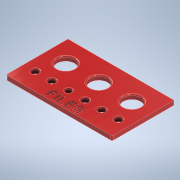
# Autodesk Inventor part: plateForFileSet
Saved by Autodesk Inventor 2021 (Build 250183000, 183)
## iProperties
Created: 2020-03-12
Part Number: plateForFileSet
Material: PET Plastic
Document SubType Name: Modeling
Designer: robst
Density: 1.541 g/cm^3
Appearance: Red
Author: robst
Autodesk Inventor part; units mm, degrees
ref_plane "YZ Plane" through (0, 0, 0) normal (1, 0, 0) x (0, 1, 0)
ref_plane "XZ Plane" through (0, 0, 0) normal (0, 1, 0) x (-1, 0, 0)
ref_plane "XY Plane" through (0, 0, 0) normal (0, 0, 1) x (1, 0, 0)
sketch "Sketch1" plane through (0, 0, 0) normal (0, 1, 0) x (-1, 0, 0)
  line L0 (76.2, 44.45) -> (-76.2, 44.45)
  line L1 (-76.2, 44.45) -> (-76.2, -44.45)
  line L2 (-76.2, -44.45) -> (76.2, -44.45)
  line L3 (76.2, -44.45) -> (76.2, 44.45)
  line L4 (76.2, 44.45) -> (-76.2, -44.45) construction
  line L5 (-76.2, 44.45) -> (76.2, -44.45) construction
  point P0 (0, 0)
  dimension "depth" = 88.9
  dimension "width" = 152.4
  constraints: 12 end point, 2 midpoint, 2 parallel, 1 horizontal, 1 perpendicular
  measures "depth" distance of L2.end L0.start
  measures "width" distance of L1.end L2.end
extrude "Extrusion1" add sketch "Sketch1" against normal blind 6.35
sketch "Sketch4" plane through (0, 0, 0) normal (0, 1, 0) x (1, 0, 0)
  line L0 (-76.2, -44.45) -> (-76.2, 44.45) construction
  line L1 (-76.2, -19.05) -> (76.2, -19.05) construction
  line L2 (76.2, 44.45) -> (76.2, -44.45) construction
  line L3 (-76.2, -44.45) -> (76.2, -44.45) projected
  circle A0 centre (-59.8678, -19.05) radius 4.445
  circle A1 centre (-35.9192, -19.05) radius 4.445
  circle A2 centre (-11.9707, -19.05) radius 3.81
  circle A3 centre (11.9779, -19.05) radius 4.445
  circle A4 centre (35.9265, -19.05) radius 4.445
  line L4 (-76.2, 12.7) -> (76.2, 12.7) construction
  circle A5 centre (-47.625, 12.7) radius 12.7
  circle A6 centre (0, 12.7) radius 12.7
  circle A7 centre (47.625, 12.7) radius 12.7
  circle A8 centre (59.8751, -19.05) radius 4.445
  line L5 (64.3201, -19.05) -> (64.3201, -9.3283) construction
  point P0 (0, 0)
  dimension "file6Hole" = 8.89
  dimension "d16" = 25.4
  dimension "file1Hole" = 8.89
  dimension "gap0" = 11.8872
  dimension "file2Hole" = 8.89
  dimension "gap1" = 23.9486
  dimension "file3Hole" = 7.62
  dimension "gap2" = 23.9486
  dimension "gap3" = 23.9486
  dimension "gap4" = 23.9486
  dimension "file4Hole" = 8.89
  dimension "file5Hole" = 8.89
  dimension "frontToBackRowGap" = 31.75
  dimension "file7Hole" = 25.4
  dimension "file8Hole" = 25.4
  dimension "gap7" = 47.625
  dimension "file9Hole" = 25.4
  dimension "gap8" = 47.625
  dimension "gap6" = 28.575
  dimension "d53" = 28.575
  dimension "file6Gap" = 23.9486
  dimension "d57" = 11.8799
  constraints: 8 centre point, 6 point on line, 4 end point, 2 vertical, 1 horizontal alignment, 1 midpoint, 1 perpendicular, 12 other
  measures "file1Hole" diameter of A0
  measures "gap0" distance edge to line of A0 L0
  measures "file2Hole" diameter of A1
  measures "gap1" distance of A1.centre A0.centre
  measures "file3Hole" diameter of A2
  measures "gap2" distance of A2.centre A1.centre
  measures "gap3" distance of A3.centre A2.centre
  measures "gap4" distance of A4.centre A3.centre
  measures "file4Hole" diameter of A3
  measures "file5Hole" diameter of A4
  measures "file7Hole" diameter of A5
  measures "file8Hole" diameter of A6
  measures "gap7" distance of A6.centre A5.centre
  measures "file9Hole" diameter of A7
  measures "gap8" distance of A7.centre A6.centre
  measures "gap6" distance from line of A5.centre L0
  measures "d53" distance from line of A7.centre L2
  measures "file6Gap" distance of point (59.875, -19.05) A4.centre
  measures "d57" distance of point (76.2, -19.05) L5.start
extrude "Extrusion3" cut sketch "Sketch4" against normal through all
sketch "Sketch8" plane through (0, 0, 0) normal (0, 1, 0) x (1, 0, 0)
  line L0 (76.2, -44.45) -> (-76.2, -44.45) construction
  line L1 (-76.2, -44.45) -> (76.2, -44.45) construction
  line L2 (-23.8464, -41.91) -> (-23.8464, -29.21)
  line L3 (-23.8464, -29.21) -> (-15.1248, -29.21)
  line L4 (-15.1248, -29.21) -> (-15.1248, -31.3589)
  line L5 (-15.1248, -31.3589) -> (-21.2812, -31.3589)
  line L6 (-21.2812, -31.3589) -> (-21.2812, -34.3597)
  line L7 (-21.2812, -34.3597) -> (-15.967, -34.3597)
  line L8 (-15.967, -34.3597) -> (-15.967, -36.5086)
  line L9 (-15.967, -36.5086) -> (-21.2812, -36.5086)
  line L10 (-21.2812, -36.5086) -> (-21.2812, -41.91)
  line L11 (-21.2812, -41.91) -> (-23.8464, -41.91)
  line L12 (-13.092, -41.91) -> (-13.092, -29.21)
  line L13 (-13.092, -29.21) -> (-10.5269, -29.21)
  line L14 (-10.5269, -29.21) -> (-10.5269, -41.91)
  line L15 (-10.5269, -41.91) -> (-13.092, -41.91)
  line L16 (-8.0101, -41.91) -> (-8.0101, -29.3165)
  line L17 (-8.0101, -29.3165) -> (-5.4449, -29.3165)
  line L18 (-5.4449, -29.3165) -> (-5.4449, -39.7611)
  line L19 (-5.4449, -39.7611) -> (0.9341, -39.7611)
  line L20 (0.9341, -39.7611) -> (0.9341, -41.91)
  line L21 (0.9341, -41.91) -> (-8.0101, -41.91)
  line L22 (2.7636, -41.91) -> (2.7636, -29.21)
  line L23 (2.7636, -29.21) -> (12.1821, -29.21)
  line L24 (12.1821, -29.21) -> (12.1821, -31.3589)
  line L25 (12.1821, -31.3589) -> (5.3288, -31.3589)
  line L26 (5.3288, -31.3589) -> (5.3288, -34.1758)
  line L27 (5.3288, -34.1758) -> (11.7078, -34.1758)
  line L28 (11.7078, -34.1758) -> (11.7078, -36.3247)
  line L29 (11.7078, -36.3247) -> (5.3288, -36.3247)
  line L30 (5.3288, -36.3247) -> (5.3288, -39.7611)
  line L31 (5.3288, -39.7611) -> (12.4241, -39.7611)
  line L32 (12.4241, -39.7611) -> (12.4241, -41.91)
  line L33 (12.4241, -41.91) -> (2.7636, -41.91)
  line L34 (13.9439, -37.767) -> (16.4413, -37.525)
  spline S0 degree 2 poles (16.4413, -37.525) (16.6639, -38.7834) (18.0481, -39.9643) (19.2097, -39.9643) knots 0 0 0 1 2 2 2
  spline S1 degree 2 poles (19.2097, -39.9643) (20.4487, -39.9643) (21.7071, -38.9189) (21.7071, -38.2123) knots 0 0 0 1 2 2 2
  spline S2 degree 2 poles (21.7071, -38.2123) (21.7071, -37.7573) (21.1747, -37.1281) (20.5165, -36.8958) knots 0 0 0 1 2 2 2
  spline S3 degree 2 poles (20.5165, -36.8958) (20.0712, -36.7409) (18.4644, -36.3441) knots 0 0 0 1 1 1
  spline S4 degree 2 poles (18.4644, -36.3441) (16.4026, -35.831) (15.5701, -35.0857) knots 0 0 0 1 1 1
  spline S5 degree 2 poles (15.5701, -35.0857) (14.3988, -34.0403) (14.3988, -32.5399) knots 0 0 0 1 1 1
  spline S6 degree 2 poles (14.3988, -32.5399) (14.3988, -31.5622) (15.5023, -29.8779) (17.5738, -28.997) (19.0355, -28.997) knots 0 0 0 1 2 3 3 3
  spline S7 degree 2 poles (19.0355, -28.997) (21.4264, -28.997) (23.8464, -31.0879) (23.9045, -32.84) knots 0 0 0 1 2 2 2
  line L35 (23.9045, -32.84) -> (21.3393, -32.9561)
  spline S8 degree 2 poles (21.3393, -32.9561) (21.1747, -31.9784) (20.0906, -31.1169) (19.0064, -31.1169) knots 0 0 0 1 2 2 2
  spline S9 degree 2 poles (19.0064, -31.1169) (17.8836, -31.1169) (17.2544, -31.5719) knots 0 0 0 1 1 1
  spline S10 degree 2 poles (17.2544, -31.5719) (16.8478, -31.872) (16.8478, -32.3656) knots 0 0 0 1 1 1
  spline S11 degree 2 poles (16.8478, -32.3656) (16.8478, -32.8109) (17.2253, -33.14) knots 0 0 0 1 1 1
  spline S12 degree 2 poles (17.2253, -33.14) (17.719, -33.5466) (21.4651, -34.4275) (23.2559, -35.3664) (24.2723, -37.0023) (24.2723, -38.2123) knots 0 0 0 1 2 3 4 4 4
  spline S13 degree 2 poles (24.2723, -38.2123) (24.2723, -39.2964) (23.0623, -41.2034) (20.8456, -42.1326) (19.1904, -42.1326) knots 0 0 0 1 2 3 3 3
  spline S14 degree 2 poles (19.1904, -42.1326) (16.7801, -42.1326) (14.1955, -39.9063) (13.9439, -37.767) knots 0 0 0 1 2 2 2
  point P0 (0, 0)
  constraints: 2 end point, 1 collinear, 1 horizontal
extrude "Extrusion5" cut sketch "Sketch8" against normal blind 2.54
fillet "Fillet5" radius 1.5875 9 edges at (-60.325, 0, -12.7) (-12.7, 0, -12.7) (34.925, 0, -12.7) (55.4301, 0, 19.05) (31.4815, 0, 19.05) (7.5329, 0, 19.05) (-15.7807, 0, 19.05) (-40.3642, 0, 19.05) (-64.3128, 0, 19.05)
fillet "Fillet6" radius 1.5875 2 edges at (-76.2, -3.175, 44.45) (76.2, -3.175, 44.45)
equation "\"frontGapBetweenHoles\" = 8.70857"
equation "\"backGapBetweenHoles\" = 9.525"
equation "\"centerLineForFrontText\" = 8.3185"
equation "\"centerLineForBackText\" = 40.64"
equation "\"largeFileHoleDiameter\" = 25.4"
equation "\"smallFileHoleDiameter\" = 8.89"
equation "\"filesInBackRow\" = 76.2"
equation "\"filesInFrontRow\" = 177.8"
equation "\"largeFileHandleDiameter\" = 38.1"
equation "\"smallFileHandleDiameter\" = 15.24"
body "Solid1"
